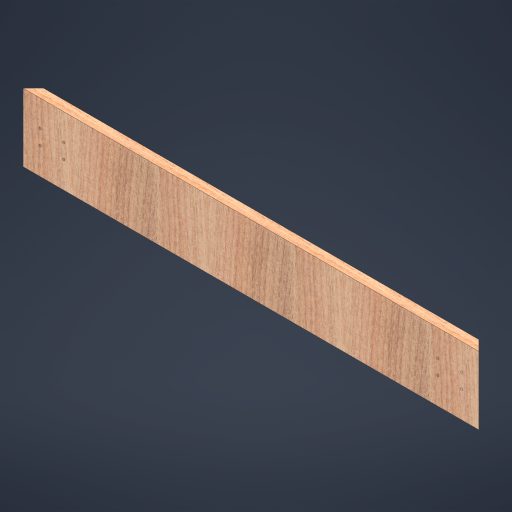
# Autodesk Inventor part: BUMP_001_Wood1
Saved by Autodesk Inventor 2024.2 (Build 282272000, 272)
## iProperties
Created: 2024-08-06
Part Number: BUMP_001_Wood1
Material: Wood (Birch)
Document SubType Name: Modeling
Designer: Bryan
Density: 0.55 g/cm^3
Appearance: Birch - Natural Polished
Author: Bryan
Autodesk Inventor part; units mm, degrees
ref_plane "YZ Plane" through (0, 0, 0) normal (1, 0, 0) x (0, 1, 0)
ref_plane "XZ Plane" through (0, 0, 0) normal (0, 1, 0) x (-1, 0, 0)
ref_plane "XY Plane" through (0, 0, 0) normal (0, 0, 1) x (1, 0, 0)
sketch "Sketch1" plane through (0, 0, 0) normal (0, 1, 0) x (-1, 0, 0)
  line L0 (-406.4, -406.4) -> (406.4, -406.4) construction
  line L1 (406.4, -406.4) -> (406.4, 406.4) construction
  line L2 (406.4, 406.4) -> (-406.4, 406.4)
  line L3 (-406.4, 406.4) -> (-406.4, -406.4) construction
  line L4 (-406.4, -406.4) -> (406.4, 406.4) construction
  line L5 (406.4, -406.4) -> (-406.4, 406.4) construction
  line L6 (425.45, 425.45) -> (425.45, -425.45) construction
  line L7 (425.45, -425.45) -> (-425.45, -425.45) construction
  line L8 (-425.45, -425.45) -> (-425.45, 425.45) construction
  line L9 (-425.45, 425.45) -> (425.45, 425.45)
  line L10 (425.45, 425.45) -> (406.4, 406.4)
  line L11 (-406.4, 406.4) -> (-425.45, 425.45)
  point P0 (0, 0)
  dimension "d0" = 812.8
  dimension "d1" = 812.8
  dimension "d2" = 19.05
  constraints: 24 end point, 4 parallel, 2 midpoint, 2 perpendicular, 1 horizontal, 3 other
  measures "d0" distance of L2.end L1.end
  measures "d1" distance of L1.end L0.end
  measures "d2" distance between parallel lines of L1 L6
extrude "Extrusion1" add sketch "Sketch1" along normal blind 127
sketch "Sketch2" plane through (406.4, 0, 406.4) normal (0, 0, -1) x (-1, 0, 0)
  line L0 (0, 0) -> (812.8, 0) projected
  line L1 (812.8, 0) -> (812.8, 127) projected
  line L2 (0, 127) -> (812.8, 127) projected
  line L3 (0, 0) -> (0, 127) projected
  line L4 (0, 0) -> (0, 127) projected
  circle A0 centre (12.7, 77.2583) radius 1.905
  line L5 (0, 77.2583) -> (12.7, 77.2583) construction
  circle A1 centre (57.15, 77.2583) radius 1.905
  circle A2 centre (101.6, 77.2583) radius 1.905 construction
  circle A3 centre (12.7, 49.7417) radius 1.905
  circle A4 centre (57.15, 49.7417) radius 1.905
  circle A5 centre (101.6, 49.7417) radius 1.905 construction
  line L6 (406.4, 127) -> (406.4, 0) construction
  circle A6 centre (800.1, 77.2583) radius 1.905
  circle A7 centre (755.65, 77.2583) radius 1.905
  circle A8 centre (711.2, 77.2583) radius 1.905 construction
  circle A9 centre (800.1, 49.7417) radius 1.905
  circle A10 centre (755.65, 49.7417) radius 1.905
  circle A11 centre (711.2, 49.7417) radius 1.905 construction
  line L7 (12.7, 77.2583) -> (12.7, 49.7417) construction
  line L8 (-19.05, 0) -> (-19.05, 127) projected
  point P0 (0, 63.5)
  point P1 (0, 63.5)
  point P2 (12.7, 63.5)
  dimension "d9" = 3.81
  dimension "d11" = 127
  dimension "d16" = 44.45
  dimension "d19" = 27.5167
  dimension "d29" = 63.5
  dimension "d30" = 31.75
  constraints: 12 centre point, 7 symmetric about line, 6 end point, 4 midpoint, 3 vertical, 2 coincident, 2 horizontal, 1 point on line, 16 other
  measures "d9" diameter of A0
  measures "d11" distance of L0.start L2.start
  measures "d16" distance of A0.centre A1.centre
  measures "d19" distance of A0.centre L7.end
  measures "d29" distance from line of L2 point (12.7, 63.5)
  measures "d30" distance between parallel lines of L8 L7
extrude "Extrusion2" cut sketch "Sketch2" against normal blind 127 contours A0 | A1 | A3 | A4 | A6 | A7 | A9 | A10
body "Solid1"
